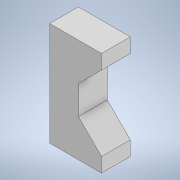
# Autodesk Inventor part: V_Holder
Saved by Autodesk Inventor 2021 (Build 250183000, 183)
## iProperties
Created: 2021-02-26
Part Number: V_Holder
Material: Generic
Document SubType Name: Modeling
Designer: Viktor
Density: 1 g/cm^3
Appearance: Default
Author: Viktor
## iProperties of the stored document _3DPrint.ipt
Created: 2021-02-26
Part Number: _3DPrint
Material: Generic
Document SubType Name: Modeling
Designer: Viktor
Density: 1 g/cm^3
Appearance: Default
Author: Viktor
Autodesk Inventor part; units mm, degrees
ref_plane "YZ Plane" through (0, 0, 0) normal (1, 0, 0) x (0, 1, 0)
ref_plane "XZ Plane" through (0, 0, 0) normal (0, 1, 0) x (-1, 0, 0)
ref_plane "XY Plane" through (0, 0, 0) normal (0, 0, 1) x (1, 0, 0)
sketch "Sketch1" plane through (0, 0, 0) normal (0, 0, 1) x (1, 0, 0)
  line L0 (-2.5, -18) -> (2.5, -18)
  line L1 (2.5, -18) -> (2.5, 18)
  line L2 (2.5, 18) -> (-2.5, 18)
  line L3 (-2.5, 18) -> (-2.5, -18)
  line L4 (-2.5, -18) -> (2.5, 18) construction
  line L5 (2.5, -18) -> (-2.5, 18) construction
  line L6 (2.5, 0) -> (20.5, 18)
  line L7 (20.5, 18) -> (2.5, 18)
  line L8 (-7.1, 0) -> (25.1, 0) projected
  line L9 (2.5, 0) -> (20.5, -18)
  line L10 (20.5, -18) -> (2.5, -18)
  line L11 (15.5, 18) -> (15.5, 13)
  line L12 (15.5, -18) -> (15.5, -13)
  line L13 (7.5, 5) -> (7.5, -5)
  point P0 (0, 0)
  point P1 (15.5, -13)
  dimension "d1" = 5
  dimension "d3" = 45
  dimension "d4" = 18
  dimension "d5" = 5
  dimension "d6" = 5
  constraints: 26 end point, 4 point on line, 3 midpoint, 3 symmetric about line, 2 horizontal, 2 parallel, 2 perpendicular, 1 vertical
  measures "d1" distance between parallel lines of L3 L1
  measures "d3" angle of L1 L6
  measures "d4" distance from line of point (0, 0) L7
  measures "d5" distance from line of L6.end L11
  measures "d6" distance from line of L6.start L13
extrude "Extrusion1" add sketch "Sketch1" along normal blind 10 contours L3 L8 L1 L0 | L1 L9 L12 L10 | L3 L2 L1 L8 | L1 L7 L11 L6 | L6 L13 L8 | L8 L13 L9
body "Solid1"
